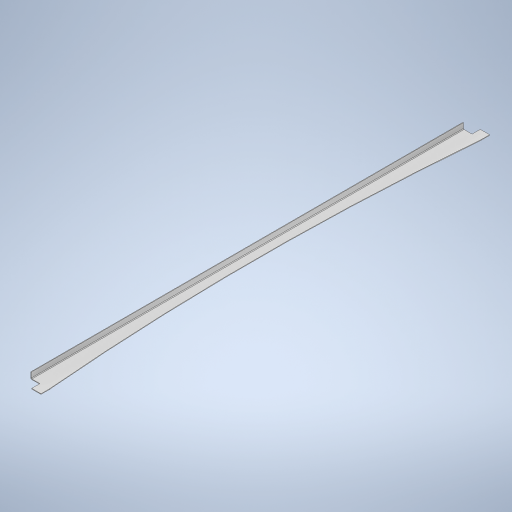
# Autodesk Inventor part: МОО 040 шпангоут борт 1
Saved by Autodesk Inventor 2024.2 (Build 282272000, 272)
## iProperties
Created: 2024-04-28
Part Number: МОО 040 шпангоут борт 1
Material: Generic
Document SubType Name: Sheet Metal
Designer: admin
Density: 1 g/cm^3
Sheet Metal Rule: Default_mm
Appearance: Default
Author: admin
Autodesk Inventor part; units mm, degrees
ref_plane "YZ Plane" through (0, 0, 0) normal (1, 0, 0) x (0, 1, 0)
ref_plane "XZ Plane" through (0, 0, 0) normal (0, 1, 0) x (-1, 0, 0)
ref_plane "XY Plane" through (0, 0, 0) normal (0, 0, 1) x (1, 0, 0)
sketch "Sketch1" plane through (0, 0, 0) normal (0, 0, 1) x (1, 0, 0)
  line L0 (0, 1050) -> (45, 1050)
  line L1 (45, 1050) -> (45, -1050) construction
  line L2 (45, -1050) -> (0, -1050)
  line L3 (0, -1050) -> (0, 1050) construction
  line L4 (0, 1050) -> (-45, 1050)
  line L5 (-45, 1050) -> (-45, -1050)
  line L6 (-45, -1050) -> (0, -1050)
  arc A0 (0, 1050) -> (0, -1050) centre (12227.5, 0) ccw construction
  arc A1 (45, 1050) -> (45, -1050) centre (12272.5, 0) ccw
  line L7 (0, 1050) -> (0, 1090)
  line L8 (0, 1090) -> (45, 1090)
  line L9 (45, 1090) -> (45, 1050)
  line L10 (0, -1050) -> (0, -1090)
  line L11 (0, -1090) -> (45, -1090)
  line L12 (45, -1090) -> (45, -1050)
  line L13 (45, 1050) -> (27.8917, 850.77) construction
  point P0 (0, 0)
  point P1 (0, 0)
  dimension "d0" = 2100
  dimension "d1" = 45
  dimension "d2" = 40
  dimension "d3" = 4.908
  measures "d0" distance of L5.start L6.start
  measures "d1" distance of L3.end L5.start
  measures "d2" distance of L9.start L1.start
  measures "d3" angle of L1 L13
extrude "Plate1" add sketch "Sketch1" along normal blind 3
sketch "Sketch2" plane through (-42, -1050, 0) normal (-1, 0, 0) x (0, -1, 0)
  line L0 (-2100, 0) -> (0, 0)
  line L1 (0, 0) -> (0, 30)
  line L2 (0, 30) -> (-2100, 30)
  line L3 (-2100, 30) -> (-2100, 0)
  constraints: 6 end point, 1 horizontal, 1 perpendicular, 1 vertical
edge flange "Flange1" height 30 angle 90 thickness 3 bend radius 3 thickness toward (-1, 0, 0) relief straight relief width 3 relief depth 1.5 edges at (-45, 0, 3) wall of the first edge with corners at (-42, 1050, 0) (-42, -1050, 0) (-42, -1050, 30) (-42, 1050, 30)
bend "Bend1"
corner "Corner1"
equation "\"d2\" = d4"
equation "\"d5\" = Thickness"
equation "\"d6\" = BendReliefWidth"
equation "\"d7\" = BendReliefDepth"
equation "\"d8\" = MinimumRemnant"
equation "\"d9\" = TransitionRadius"
equation "\"d12\" = BendRadius"
equation "\"d13\" = CornerReliefSize"
equation "\"d14\" = GapSize"
equation "\"d15\" = JacobiRadiusSize"
equation "\"BendRadius\" = Thickness"
equation "\"BendReliefWidth\" = Thickness"
equation "\"BendReliefDepth\" = 0.5 * Thickness"
equation "\"CornerReliefSize\" = 4 * Thickness"
equation "\"MinimumRemnant\" = 2 * Thickness"
equation "\"TransitionRadius\" = BendRadius"
equation "\"JacobiRadiusSize\" = BendRadius"
equation "\"GapSize\" = Thickness"
equation "\"d4\" = 40"
equation "\"Thickness\" = 3"
body "Solid1"
